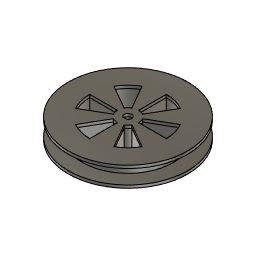
MotorReel v2 (Autodesk Fusion 360 design; units mm, degrees)
Autodesk Fusion 360 part; units mm, degrees
note: some values were not read from the file. Set by a fixed rule: which sketch regions a step uses.
sketch "Sketch1" plane through (0, 0, 0) normal (0, 0, 1) x (1, 0, 0)
  circle A0 centre (0, 0) radius 31.831
  circle A1 centre (0, 0) radius 41.831
  circle A2 centre (0, 0) radius 2.6
  line L0 (-1.533, -2.1) -> (1.533, -2.1)
  line L1 (0, 0) -> (0, 3.1) construction
  line L2 (0, 3.1) -> (0, 2.6) construction
  line L3 (2.9, 2.6) -> (0, 2.6) construction
  circle A3 centre (0, 0) radius 7.5
  circle A4 centre (0, 0) radius 26.831
  line L4 (0, -7.5) -> (0, -26.831)
  line L5 (3.75, -6.4952) -> (13.4155, -23.2363)
  line L6 (6.4952, -3.75) -> (23.2363, -13.4155)
  line L7 (7.5, 0) -> (26.831, 0)
  line L8 (6.4952, 3.75) -> (23.2363, 13.4155)
  line L9 (3.75, 6.4952) -> (13.4155, 23.2363)
  line L10 (0, 7.5) -> (0, 26.831)
  line L11 (-3.75, 6.4952) -> (-13.4155, 23.2363)
  line L12 (-6.4952, 3.75) -> (-23.2363, 13.4155)
  line L13 (-7.5, 0) -> (-26.831, 0)
  line L14 (-6.4952, -3.75) -> (-23.2363, -13.4155)
  line L15 (-3.75, -6.4952) -> (-13.4155, -23.2363)
  circle A5 centre (0, 33.331) radius 1.5
  line L16 (0, 0) -> (0, 44.6425) construction
  circle A6 centre (-5, 32.9538) radius 1.5
  dimension "d2" = 63.662
  dimension "d3" = 10
  dimension "d12" = 5.2
  dimension "d13" = 2.1
  dimension "d16" = 15
  dimension "d17" = -5
  dimension "d19" = 360
  dimension "d22" = 3
  dimension "d23" = 3
  dimension "d24" = 5
  constraint coincident A0.centre A1.centre
  constraint concentric A0 A2
  constraint coincident A2 L0.start
  constraint coincident A2 L0.end
  constraint horizontal L0
  constraint vertical L1
  constraint coincident L1 L2.end
  constraint coincident A2 L2.end
  constraint perpendicular L1 L3
  constraint concentric A2 A3
  constraint coincident A3 L4.start
  constraint coincident A4 L4.end
  constraint vertical L4
  constraint tangent A0 A5
  constraint parallel L1 L16
  constraint coincident A5.centre L16
  constraint tangent A0 A6
  measures "d2" diameter of A0
  measures "d12" diameter of A2
  measures "d13" distance of A0.centre L0
  measures "d16" diameter of A3
  measures "d22" diameter of A5
  measures "d23" diameter of A6
  measures "d24" horizontal distance of A5.centre A6.centre
extrude "Extrude1" add sketch "Sketch1" along normal blind 2 contours A6 | A5 | A1 makes body 1
extrude "Extrude2" add sketch "Sketch1" along normal blind 12 contours A0 | A2 L0 | A2 L0 | A3 | A3 A4 L6 L7 | A3 A4 L7 L8 | A3 A4 L8 L9 | A3 A4 L5 L6 | A3 A4 L9 L10 | A3 A4 L4 L5 | A3 A4 L10 L11 | A3 A4 L4 L15 | A3 A4 L11 L12 | A3 A4 L14 L15 | A3 A4 L12 L13 | A3 A4 L13 L14 bodies 1
sketch "Sketch2" plane through (0, 0, 12) normal (0, 0, 1) x (-1, 0, 0)
  circle A0 centre (0, 0) radius 31.831
  circle A1 centre (0, 0) radius 41.831
  dimension "d8" = 10
extrude "Extrude3" add sketch "Sketch2" along normal blind 2 separate body contours A0 | A1 makes body 2
extrude "Extrude4" cut sketch "Sketch1" along normal blind 14 contours A2 L0 picked at (0.7232, -0.5742) bodies 1 2
extrude "Extrude5" cut sketch "Sketch1" along normal blind 14 contours A3 A4 L7 L8 | A3 A4 L5 L6 | A3 A4 L9 L10 | A3 A4 L4 L15 | A3 A4 L11 L12 | A3 A4 L13 L14 bodies 1 2
extrude "Extrude6" cut sketch "Sketch1" along normal blind 2 contours A6 | A5 bodies 1
equation "circ = 63.662 mm"
equation "d2 = circ"
equation "d6 = 2 mm + 10 mm"
equation "MotorShaftTolerance = 0.2 mm"
equation "d12 = 5 mm + MotorShaftTolerance"
equation "d13 = 2.5 mm - 0.4 mm"
